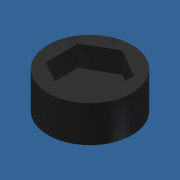
# Autodesk Inventor part: M5_encoderMagnet
Saved by Autodesk Inventor 2014 SP2 (Build 180246200, 246)
## iProperties
Created: 2015-01-28
Part Number: M5_encoderMagnet
Material: ABS-Kunststoff - Schwarz
Document SubType Name: Modeling
Designer: 4ndreas
Density: 1.06 g/cm^3
Appearance: Glatt - weiß(2)
Author: 4ndreas
Autodesk Inventor part; units mm, degrees
ref_plane "YZ Plane" through (0, 0, 0) normal (1, 0, 0) x (0, 1, 0)
ref_plane "XZ Plane" through (0, 0, 0) normal (0, 1, 0) x (-1, 0, 0)
ref_plane "XY Plane" through (0, 0, 0) normal (0, 0, 1) x (1, 0, 0)
sketch "Skizze1" plane through (0, 0, 0) normal (0, 0, 1) x (1, 0, 0)
  circle A0 centre (0, 0) radius 6
  circle A1 centre (0, 0) radius 3.05
  dimension "d0" = 6.1
  dimension "d1" = 12
  constraints: 2 centre point, 2 coincident
  measures "d0" diameter of A1
  measures "d1" diameter of A0
extrude "Extrusion1" add sketch "Skizze1" along normal blind 2
sketch "Skizze2" plane through (0, 0, 2) normal (0, 0, 1) x (1, 0, 0)
  circle A0 centre (0, 0) radius 6 projected
extrude "Extrusion2" add sketch "Skizze2" along normal blind 0.2
sketch "Skizze3" plane through (0, 0, 2.2) normal (0, 0, 1) x (1, 0, 0)
  circle A0 centre (0, 0) radius 6 projected
  line L0 (0, 4.6188) -> (4, 2.3094)
  line L1 (4, 2.3094) -> (4, -2.3094)
  line L2 (4, -2.3094) -> (0, -4.6188)
  line L3 (0, -4.6188) -> (-4, -2.3094)
  line L4 (-4, -2.3094) -> (-4, 2.3094)
  line L5 (-4, 2.3094) -> (0, 4.6188)
  dimension "d6" = 8
  constraints: 12 end point, 1 coincident, 1 vertical, 13 other
  measures "d6" distance between parallel lines of L1 L4
extrude "Extrusion3" add sketch "Skizze3" along normal blind 3
